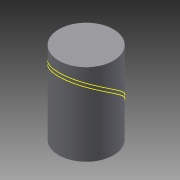
# Autodesk Inventor part: newDrumCam
Saved by Autodesk Inventor 2015 (Build 190159000, 159)
## iProperties
Created: 2015-04-29
Part Number: newDrumCam
Material: Generic
Document SubType Name: Modeling
Designer: WASHHSST
Density: 1 g/cm^3
Appearance: Default
Author: WASHHSST
Autodesk Inventor part; units mm, degrees
ref_plane "YZ Plane" through (0, 0, 0) normal (1, 0, 0) x (0, 1, 0)
ref_plane "XZ Plane" through (0, 0, 0) normal (0, 1, 0) x (-1, 0, 0)
sketch "Sketch1" plane through (0, 0, 0) normal (0, 1, 0) x (-1, 0, 0)
  circle A0 centre (0, 0) radius 101.6
  dimension "d0" = 203.2
  constraints: 1 centre point, 1 coincident
  measures "d0" diameter of A0
extrude "Extrusion1" add sketch "Sketch1" along normal blind 304.8
ref_plane "Work Plane2" through (0, 0, 101.6) normal (0, 0, 1) x (1, 0, 0)
sketch "Sketch3" plane through (0, 0, 101.6) normal (0, 0, 1) x (1, 0, 0)
  line L0 (-319.1858, 50.8) -> (319.1858, 50.8) construction
  line L1 (-319.1858, 254) -> (319.1858, 254) construction
  line L2 (-319.1858, 38.1) -> (319.1858, 38.1) construction
  line L3 (-319.1858, 266.7) -> (319.1858, 266.7) construction
  spline S0 degree 2 poles (-319.1858, 38.1) (0, 469.9) (319.1858, 38.1) knots 0 0 0 1 1 1
  spline S1 degree 2 poles (319.1858, 50.8) (0, 482.6) (-319.1858, 50.8) knots 0 0 0 1 1 1
  line L4 (-319.1858, 50.8) -> (-319.1858, 38.1)
  line L5 (319.1858, 50.8) -> (319.1858, 38.1)
  line L6 (-101.6, 0) -> (-101.6, 304.8) projected
  point P0 (0, 0)
  point P1 (0, 254)
  point P2 (0, 266.7)
  dimension "d3" = 638.3716
  dimension "d4" = 50.8
  dimension "d5" = 319.1858
  dimension "d6" = 254
  dimension "d7" = 12.7
  dimension "d8" = 12.7
  dimension "d9" = 12.7
  dimension "d10" = 203.2
  dimension "d11" = 12.7
  dimension "d12" = 12.7
  constraints: 12 end point, 3 parallel, 2 midpoint, 1 horizontal, 1 vertical, 6 other
  measures "d3" distance of L0.start L0.end
  measures "d4" distance from line of L0 point (0, 0)
  measures "d5" horizontal distance of L0.start point (0, 0)
  measures "d6" distance from line of L1 point (0, 0)
  measures "d7" distance between parallel lines of L0 L2
  measures "d8" distance between parallel lines of L1 L3
  measures "d9" distance of L0.end L2.end
  measures "d10" distance from line of L0 point (0, 254)
  measures "d11" distance of point (0, 254) point (0, 266.7)
  measures "d12" distance from line of L3 point (0, 254)
sketch3d "3D Sketch1"
body "Solid1"
